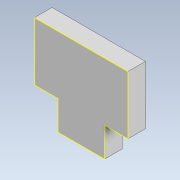
# Autodesk Inventor part: bracket_2
Saved by Autodesk Inventor 2022 (Build 260153000, 153)
## iProperties
Created: 2023-05-02
Part Number: bracket_2
Material: 一般
Document SubType Name: Modeling
Designer: JOU
Density: 1 g/cm^3
Appearance: 預設
Author: JOU
Autodesk Inventor part; units mm, degrees
ref_plane "YZ Plane" through (0, 0, 0) normal (1, 0, 0) x (0, 1, 0)
ref_plane "XZ Plane" through (0, 0, 0) normal (0, 1, 0) x (-1, 0, 0)
ref_plane "XY Plane" through (0, 0, 0) normal (0, 0, 1) x (1, 0, 0)
sketch "草圖1" plane through (0, 0, 0) normal (0, 0, 1) x (1, 0, 0)
  line L0 (0, 0) -> (8, 0)
  line L1 (8, 0) -> (8, 5)
  line L2 (8, 5) -> (0, 5)
  line L3 (0, 5) -> (0, 0)
  line L4 (-4, 15) -> (12, 15)
  line L5 (12, 15) -> (12, 5)
  line L6 (12, 5) -> (-4, 5)
  line L7 (-4, 5) -> (-4, 15)
  dimension "d0" = 8
  dimension "d1" = 5
  dimension "d2" = 4
  dimension "d3" = 4
  dimension "d4" = 10
  constraints: 16 end point, 4 parallel, 2 horizontal, 2 perpendicular, 1 collinear
  measures "d0" distance of L1.end L2.end
  measures "d1" distance of L0.end L1.end
  measures "d2" distance between parallel lines of L3 L7
  measures "d3" distance between parallel lines of L1 L5
  measures "d4" distance of L4.end L5.end
extrude "擠出1" add sketch "草圖1" along normal blind 3
sketch "草圖2" plane through (0, 0, 3) normal (0, 0, 1) x (1, 0, 0)
  line L0 (12, 15) -> (-4, 15) projected
  line L1 (-4, 15) -> (-4, 5) projected
  line L2 (-4, 5) -> (0, 5) projected
  line L3 (0, 5) -> (0, 0) projected
  line L4 (0, 0) -> (8, 0) projected
  line L5 (8, 0) -> (8, 5) projected
  line L6 (8, 5) -> (12, 5) projected
  line L7 (12, 5) -> (12, 15) projected
